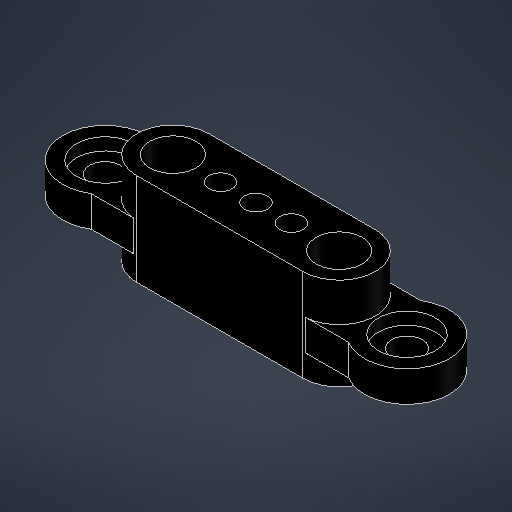
# Autodesk Inventor part: Pogo2
Saved by Autodesk Inventor 2026 (Build 300175000, 175)
## iProperties
Created: 2025-04-17
Part Number: Pogo2
Material: Nylon 6/6
Document SubType Name: Modeling
Designer: ct_vi
Density: 1.13 g/cm^3
Appearance: Nylon 6
Author: ct_vi
Autodesk Inventor part; units mm, degrees
ref_plane "YZ Plane" through (0, 0, 0) normal (1, 0, 0) x (0, 1, 0)
ref_plane "XZ Plane" through (0, 0, 0) normal (0, 1, 0) x (-1, 0, 0)
sketch "Sketch1" plane through (0, 0, 0) normal (0, 1, 0) x (-1, 0, 0)
  line L0 (-8.55, 0) -> (-8.55, 0)
  line L1 (5.4, 2.35) -> (-5.4, 2.35)
  line L2 (-7.75, 0) -> (-7.75, 0)
  line L3 (7.75, 0) -> (7.75, 0)
  arc A0 (-5.4, 2.35) -> (-7.75, 0) centre (-5.4, 0) ccw
  arc A1 (-7.75, 0) -> (-5.4, -2.35) centre (-5.4, 0) ccw
  arc A2 (7.75, 0) -> (5.4, 2.35) centre (5.4, 0) ccw
  arc A3 (5.4, -2.35) -> (7.75, 0) centre (5.4, 0) ccw
  circle A4 centre (5.4, 0) radius 1.5
  circle A5 centre (-5.4, 0) radius 1.5
  circle A6 centre (2.3, 0) radius 0.75
  circle A7 centre (0, 0) radius 0.75
  circle A8 centre (-2.3, 0) radius 0.75
  circle A9 centre (2.3, 0) radius 0.35
  circle A10 centre (0, 0) radius 0.35
  circle A11 centre (-2.3, 0) radius 0.45
  line L4 (-15.2366, 19.4813) -> (26.8433, 19.4813) construction
  line L5 (26.8433, 19.4813) -> (26.8433, -5.0467) construction
  line L6 (26.8433, -5.0467) -> (-15.2366, -5.0467) construction
  line L7 (-15.2366, -5.0467) -> (-15.2366, 19.4813) construction
  line L8 (-8.3717, -2.35) -> (8.3717, -2.35)
  line L9 (8.3717, 2.35) -> (-8.3717, 2.35)
  circle A12 centre (2.3, 0) radius 1.05
  circle A13 centre (0, 0) radius 1.05
  circle A14 centre (-2.3, 0) radius 1.05
  point P0 (7.75, 0)
  point P1 (-5.4, -2.35)
  point P2 (5.4, -2.35)
  dimension "d5" = 2.35
  dimension "d6" = 3
  dimension "d7" = 3
  dimension "d10" = 1.5
  dimension "d11" = 4.6
  dimension "d14" = 0.9
  dimension "d201" = 2.1
  dimension "d202" = 2.1
  dimension "d203" = 2.1
  dimension "d204" = 1.5
  dimension "d205" = 1.5
  constraints: 15 centre point, 12 end point, 8 point on circle, 6 tangent, 5 coincident, 3 equal radius, 2 horizontal, 2 parallel, 1 perpendicular, 2 other
  measures "d5" radius of A0
  measures "d6" diameter of A4
  measures "d7" diameter of A5
  measures "d10" diameter of A8
  measures "d11" distance of A8.centre A6.centre
  measures "d14" diameter of A11
  measures "d201" diameter of A12
  measures "d202" diameter of A13
  measures "d203" diameter of A14
  measures "d204" diameter of A7
  measures "d205" diameter of A6
extrude "Extrusion1" add sketch "Sketch1" along normal blind 6 contours A2 A3 L8 A1 A0 L1 | A12 | A13 | A14
ref_plane "Work Plane1" through (0, 1.5, 0) normal (0, -1, 0) x (1, 0, 0)
sketch "Sketch2" plane through (0, 1.5, 0) normal (0, -1, 0) x (1, 0, 0)
  line L0 (0, 0) -> (9.8, 0)
  circle A0 centre (9.8, 0) radius 1
  circle A1 centre (9.8, 0) radius 1.85
  circle A2 centre (9.8, 0) radius 2.75
  line L1 (-8.3604, 2.3431) -> (8.3604, 2.3431)
  line L2 (8.3604, -2.3431) -> (-8.3604, -2.3431)
  line L3 (-8.1293, 2.1844) -> (8.1293, -2.1844) construction
  line L4 (8.1293, 2.1844) -> (-8.7202, -2.3431) construction
  line L5 (0, 0) -> (-9.8, 0)
  circle A3 centre (-9.8, 0) radius 1
  circle A4 centre (-9.8, 0) radius 1.85
  circle A5 centre (-9.8, 0) radius 2.75
  dimension "d119" = 9.8
  dimension "d120" = 2
  dimension "d121" = 3.7
  dimension "d122" = 5.5
  dimension "d126" = 9.8
  dimension "d127" = 2
  dimension "d128" = 3.7
  dimension "d130" = 5.5
  constraints: 12 end point, 7 point on circle, 6 centre point, 6 coincident, 3 horizontal, 1 midpoint, 1 parallel, 1 point on line
  measures "d119" distance of L0.start L0.end
  measures "d120" diameter of A0
  measures "d121" diameter of A1
  measures "d122" diameter of A2
  measures "d126" distance of L0.start L5.end
  measures "d127" diameter of A3
  measures "d128" diameter of A4
  measures "d130" diameter of A5
extrude "Extrusion2" add sketch "Sketch2" against normal blind 2 contours L5 A5 L1 A2 L0 | L0 A2 L2 A5 L5
extrude "Extrusion3" add sketch "Sketch2" against normal blind 2 contours A2 | A5
extrude "Extrusion4" add sketch "Sketch2" against normal blind 1.2 contours A1 | A3 | A4
sketch "Sketch3" plane through (-5.4, 0, 2.35) normal (0, 0, 1) x (1, 0, 0)
  line L0 (-9.7661, 9.6728) -> (32.2033, 9.6728) construction
  line L1 (32.2033, 9.6728) -> (32.2033, -14.7908) construction
  line L2 (32.2033, -14.7908) -> (-9.7661, -14.7908) construction
  line L3 (-9.7661, -14.7908) -> (-9.7661, 9.6728) construction
  point P0 (5.4, 0)
  constraints: 2 other
extrude "Extrusion5" cut sketch "Sketch2" against normal through all contours A0 | A3
extrude "Extrusion6" cut sketch "Sketch1" along normal through all contours A4 | A5
extrude "Extrusion7" cut sketch "Sketch1" along normal blind 10 contours A6 | A7 | A8 | A9 | A10 | A11
extrude "Extrusion8" cut sketch "Sketch1" along normal blind 0.5 contours A12 | A13 | A14
body "Solid1"
